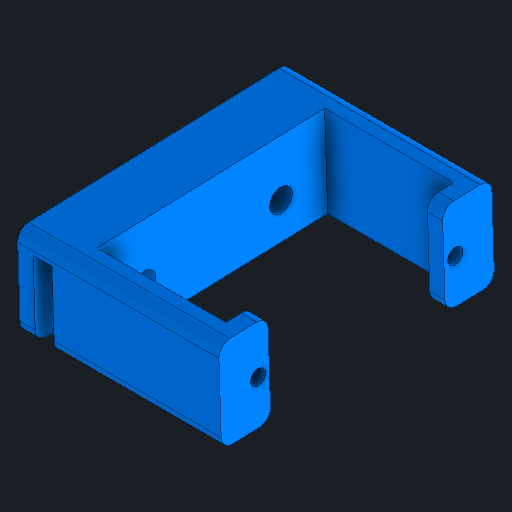
# Autodesk Inventor part: servo_mount
Saved by Autodesk Inventor 2022.2 (Build 262287010, 287A)
## iProperties
Created: 2022-03-29
Part Number: servo_mount
Material: Generic
Document SubType Name: Modeling
Designer: kardo
Density: 1 g/cm^3
Appearance: Blue Plastic
Author: kardo
Autodesk Inventor part; units mm, degrees
ref_plane "YZ Plane" through (0, 0, 0) normal (1, 0, 0) x (0, 1, 0)
ref_plane "XZ Plane" through (0, 0, 0) normal (0, 1, 0) x (-1, 0, 0)
ref_plane "XY Plane" through (0, 0, 0) normal (0, 0, 1) x (1, 0, 0)
derived "stencil_frame.ipt"
sketch "sk_servo_joint" plane through (-54.6, 0, 0) normal (1, 0, 0) x (0, 1, 0)
  line L0 (-254.1001, 19.9549) -> (9.48, 28.4869) construction
  line L1 (-363, 1541.8302) -> (-363, -1877.3857) construction
  line L2 (0, 1541.8302) -> (0, -1877.3857) construction
  line L3 (-204.8018, 21.5506) -> (-205.0153, 28.1472) construction
  line L4 (-205.0153, 28.1472) -> (-187.0247, 28.7295) construction
  line L5 (-187.0247, 28.7295) -> (-186.8112, 22.133) construction
  line L6 (-96.0723, 31.6736) -> (-99.3076, 131.6213) construction
  line L7 (-99.3076, 131.6213) -> (-199.2553, 128.386) construction
  line L8 (-199.2553, 128.386) -> (-196.02, 28.4384) construction
  line L9 (-187.0247, 28.7295) -> (-96.0723, 31.6736) construction
  point P0 (0, 0)
  point P1 (-191.0082, 43.6084)
sketch3d "sk_servo_rod"
ref_plane "plane_cowl_left" through (-54.6, 0, 0) normal (1, 0, 0) x (0, 1, 0)
derived "parameters_frame.ipt"
derived "parameters_powertrain.ipt"
sketch "sk_base" plane through (-54.6, 0, 0) normal (1, 0, 0) x (0, 1, 0)
  line L0 (-254.1001, 19.9549) -> (9.48, 28.4869) construction
  line L1 (-210.8569, 23.1556) -> (-180.8726, 24.1262)
  line L2 (-180.8726, 24.1262) -> (-181.2026, 34.3208)
  line L3 (-181.2026, 34.3208) -> (-211.1869, 33.3502)
  line L4 (-211.1869, 33.3502) -> (-210.8569, 23.1556)
  line L5 (-205.0153, 28.1472) -> (-211.0121, 27.9531) construction
  line L6 (-187.0247, 28.7295) -> (-181.0279, 28.9236) construction
  line L7 (-210.8569, 23.1556) -> (-213.8553, 23.0585)
  line L8 (-213.8553, 23.0585) -> (-214.25, 35.2521)
  line L9 (-214.25, 35.2521) -> (-178.2688, 36.4168)
  line L10 (-178.2688, 36.4168) -> (-177.8741, 24.2232)
  line L11 (-177.8741, 24.2232) -> (-180.8726, 24.1262)
  point P0 (0, 0)
  point P1 (-196.02, 28.4384)
  dimension "d1" = 18
  dimension "d2" = 1.8
  dimension "d5" = 5.4
  dimension "d6" = 30
  dimension "d8" = 2
  dimension "d9" = 3
  constraints: 22 end point, 5 parallel, 4 collinear, 4 perpendicular, 2 point on line
  measures "d1" distance of L6.start L5.start
  measures "d2" distance between parallel lines of L0 L1
  measures "d5" distance from line of point (-196.02, 28.438) L3
  measures "d6" distance between parallel lines of L2 L4
  measures "d8" distance between parallel lines of L9 L3
  measures "d9" distance between parallel lines of L8 L4
sketch "sk_side_rails" plane through (-54.6, 0, 0) normal (1, 0, 0) x (0, 1, 0)
  line L0 (-211.1869, 33.3502) -> (-210.8569, 23.1556) projected
  line L1 (-180.8726, 24.1262) -> (-181.2026, 34.3208) projected
  line L2 (-213.8553, 23.0585) -> (-210.8569, 23.1556)
  line L3 (-177.8741, 24.2232) -> (-180.8726, 24.1262)
  line L4 (-214.25, 35.2521) -> (-178.2688, 36.4168) projected
  line L5 (-213.8553, 23.0585) -> (-214.25, 35.2521) projected
  line L6 (-178.2688, 36.4168) -> (-177.8741, 24.2232) projected
  line L7 (-210.8569, 23.1556) -> (-213.8553, 23.0585) projected
  line L8 (-177.8741, 24.2232) -> (-180.8726, 24.1262) projected
  line L9 (-211.1869, 33.3502) -> (-211.2516, 35.3492)
  line L10 (-181.2026, 34.3208) -> (-181.2673, 36.3198)
  point P0 (0, 0)
  constraints: 8 end point, 2 collinear, 2 perpendicular, 2 point on line
sketch "sk_bridge" plane through (-54.6, 0, 0) normal (1, 0, 0) x (0, 1, 0)
  line L0 (-214.25, 35.2521) -> (-178.2688, 36.4168) projected
  line L1 (-181.2026, 34.3208) -> (-211.1869, 33.3502) projected
  line L2 (-214.25, 35.2521) -> (-214.1853, 33.2532)
  line L3 (-214.1853, 33.2532) -> (-211.1869, 33.3502)
  line L4 (-178.2688, 36.4168) -> (-178.2041, 34.4179)
  line L5 (-178.2041, 34.4179) -> (-181.2026, 34.3208)
  point P0 (0, 0)
  constraints: 8 end point, 2 collinear, 2 perpendicular
extrude "extrude_bridge" add sketch "sk_bridge" against normal blind 2.5
extrude "extrude_rails" add sketch "sk_side_rails" along normal blind 22
sketch "sk_backplate" plane through (-57.1, 0, 0) normal (-1, 0, 0) x (0, 0, 1)
  line L0 (36.4168, -178.2688) -> (24.2232, -177.8741) projected
  line L1 (23.1556, -210.8569) -> (24.1262, -180.8726) projected
  line L2 (24.2232, -177.8741) -> (24.1262, -180.8726) projected
  line L3 (23.1556, -210.8569) -> (23.0585, -213.8553) projected
  line L4 (23.0585, -213.8553) -> (35.2521, -214.25) projected
  line L5 (35.2521, -214.25) -> (36.4168, -178.2688) projected
  point P0 (0, 0)
extrude "extrude_backplate" add sketch "sk_backplate" along normal blind 2
sketch "sk_frontplate" plane through (-54.6, 0, 0) normal (1, 0, 0) x (0, 1, 0)
  line L0 (-213.8553, 23.0585) -> (-214.25, 35.2521) projected
  line L1 (-214.25, 35.2521) -> (-178.2688, 36.4168) projected
  line L2 (-178.2688, 36.4168) -> (-177.8741, 24.2232) projected
  line L3 (-177.8741, 24.2232) -> (-180.8726, 24.1262) projected
  line L4 (-210.8569, 23.1556) -> (-180.8726, 24.1262) projected
  line L5 (-210.8569, 23.1556) -> (-213.8553, 23.0585) projected
  point P0 (0, 0)
extrude "extrude_frontplate" add sketch "sk_frontplate" along normal blind 3
sketch "sk_drills" plane through (-54.6, 0, 0) normal (1, 0, 0) x (0, 1, 0)
  line L0 (-205.0153, 28.1472) -> (-187.0247, 28.7295) construction
  line L1 (-203.3643, 31.2333) -> (-201.5171, 28.2604)
  line L2 (-201.5171, 28.2604) -> (-203.1681, 25.1743)
  line L3 (-203.1681, 25.1743) -> (-206.6663, 25.0611)
  line L4 (-206.6663, 25.0611) -> (-208.5135, 28.0339)
  line L5 (-208.5135, 28.0339) -> (-206.8624, 31.1201)
  line L6 (-206.8624, 31.1201) -> (-203.3643, 31.2333)
  line L7 (-185.3737, 31.8156) -> (-183.5265, 28.8428)
  line L8 (-183.5265, 28.8428) -> (-185.1776, 25.7566)
  line L9 (-185.1776, 25.7566) -> (-188.6757, 25.6434)
  line L10 (-188.6757, 25.6434) -> (-190.5229, 28.6163)
  line L11 (-190.5229, 28.6163) -> (-188.8719, 31.7024)
  line L12 (-188.8719, 31.7024) -> (-185.3737, 31.8156)
  circle A0 centre (-205.0153, 28.1472) radius 1.5
  circle A1 centre (-187.0247, 28.7295) radius 1.5
  point P0 (0, 0)
  dimension "d19" = 7
  dimension "d20" = 3
  constraints: 26 end point, 4 coincident, 2 centre point, 2 point on line, 1 collinear, 1 equal radius, 26 other
  measures "d19" distance of L1.end L4.end
  measures "d20" diameter of A1
extrude "drill_hex_backplate" cut sketch "sk_drills" against normal through all contours L1 L2 L3 L4 L5 L6 | L7 L8 L9 L10 L11 L12 | A0 | A1
extrude "drill_circular_frontplate" cut sketch "sk_drills" along normal through all contours A0 | A1
sketch "sk_mounting_pads" plane through (-32.6, 0, 0) normal (1, 0, 0) x (0, 0, -1)
  line L0 (-23.1556, -210.8569) -> (-35.3492, -211.2516) projected
  line L1 (-36.3198, -181.2673) -> (-24.1262, -180.8726) projected
  line L2 (-35.3492, -211.2516) -> (-35.4624, -207.7534)
  line L3 (-35.4624, -207.7534) -> (-23.2688, -207.3587)
  line L4 (-23.2688, -207.3587) -> (-23.1556, -210.8569)
  line L5 (-36.3198, -181.2673) -> (-36.2065, -184.7654)
  line L6 (-36.2065, -184.7654) -> (-24.0129, -184.3707)
  line L7 (-24.0129, -184.3707) -> (-24.1262, -180.8726)
  point P0 (0, 0)
  dimension "d37" = 23
  constraints: 12 end point, 4 perpendicular, 2 parallel, 1 collinear
  measures "d37" distance between parallel lines of L6 L3
extrude "extrude_mounting_pads" add sketch "sk_mounting_pads" against normal blind 2
sketch "sk_pad_drills" plane through (-32.6, 0, 0) normal (1, 0, 0) x (0, 0, -1)
  line L0 (-23.2688, -207.3587) -> (-35.4624, -207.7534) construction
  line L1 (-36.2065, -184.7654) -> (-24.0129, -184.3707) construction
  line L2 (-29.0172, -209.0455) -> (-29.0658, -207.5463) construction
  line L3 (-29.8099, -184.5584) -> (-29.8584, -183.0592) construction
  line L4 (-29.0658, -207.5463) -> (-29.8099, -184.5584) construction
  line L5 (-28.1472, -205.0153) -> (-128.0948, -208.2506) construction
  line L6 (-128.0948, -208.2506) -> (-128.6772, -190.26) construction
  line L7 (-128.6772, -190.26) -> (-28.7295, -187.0247) construction
  circle A0 centre (-28.1472, -205.0153) radius 1.5 projected
  line L8 (-28.7295, -187.0247) -> (-28.1472, -205.0153) construction
  point P0 (0, 0)
  dimension "d39" = 26
  dimension "d40" = 100
  dimension "d41" = 99
  constraints: 14 end point, 3 collinear, 2 parallel, 2 perpendicular, 2 point on line
  measures "d39" distance of L2.start L3.end
  measures "d40" distance of L5.start L5.end
  measures "d41" distance between parallel lines of L6 L4
hole "drill_pads" at (-32.6, -209.0455, 29.0172) at (-32.6, -183.0592, 29.8584) direction (-1, 0, 0) diameter 2 depth 2 tip angle 118
fillet "rounding" radius 1.5 10 edges at (-45.85, -178.2688, 36.4168) (-43.6, -177.8741, 24.2232) (-58.1, -177.8741, 24.2232) (-43.6, -213.8553, 23.0585) (-45.85, -214.25, 35.2521) (-58.1, -213.8553, 23.0585) (-33.6, -207.7534, 35.4624) (-33.6, -207.3587, 23.2688) (-33.6, -184.7654, 36.2065) (-33.6, -184.3707, 24.0129)
equation "\"d5\" = 1.8 * drill_servo_mount_diam"
equation "\"d12\" = servo_pad_height_gross"
equation "\"d20\" = drill_servo_mount_diam"
equation "\"d39\" = servo_width + 2 * servo_pad_drill_outset"
equation "\"d41\" = d40 - servo_pad_drill_centerline"
equation "\"d30\" = servo_pad_drill_diam"
equation "\"servo_pad_height_gross\" = 22"
equation "\"drill_servo_mount_diam\" = 3"
equation "\"servo_width\" = 22"
equation "\"servo_pad_drill_outset\" = 2"
equation "\"servo_pad_drill_centerline\" = 1"
equation "\"servo_pad_drill_diam\" = 2"
body "Solid1"
